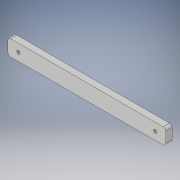
# Autodesk Inventor part: Fourbar-Coupler
Saved by Autodesk Inventor 2019 (Build 230136000, 136)
## iProperties
Created: 2021-06-06
Part Number: Fourbar-Coupler
Material: Generic
Document SubType Name: Modeling
Designer: micha
Density: 1 g/cm^3
Appearance: Default
Author: micha
Autodesk Inventor part; units mm, degrees
ref_plane "YZ Plane" through (0, 0, 0) normal (1, 0, 0) x (0, 1, 0)
ref_plane "XZ Plane" through (0, 0, 0) normal (0, 1, 0) x (-1, 0, 0)
ref_plane "XY Plane" through (0, 0, 0) normal (0, 0, 1) x (1, 0, 0)
sketch "Sketch1" plane through (0, 0, 0) normal (0, 0, 1) x (1, 0, 0)
  line L0 (0, 0) -> (300, 0)
  line L1 (300, 0) -> (300, 30)
  line L2 (300, 30) -> (0, 30)
  line L3 (0, 30) -> (0, 0)
  dimension "d0" = 300
  dimension "d1" = 30
  constraints: 8 end point, 2 parallel, 1 horizontal, 1 perpendicular
  measures "d0" distance of L2.end L1.end
  measures "d1" distance of L1.end L0.end
extrude "Extrusion1" add sketch "Sketch1" along normal blind 12
fillet "Fillet1" radius 5 1 edges at (0, 30, 6)
fillet "Fillet2" radius 5 3 edges at (300, 30, 6) (300, 0, 6) (0, 0, 6)
sketch "Sketch2" plane through (0, 0, 12) normal (0, 0, 1) x (1, 0, 0)
  line L0 (0, 25) -> (0, 5) projected
  line L1 (0, 15) -> (20, 15)
  circle A0 centre (20, 15) radius 3
  line L2 (5, 0) -> (295, 0) projected
  line L3 (150, 0) -> (150, 30)
  line L4 (295, 30) -> (5, 30) projected
  circle A1 centre (280, 15) radius 3
  point P0 (0, 0)
  dimension "d6" = 20
  dimension "d7" = 6
  constraints: 4 end point, 3 midpoint, 2 centre point, 1 coincident, 1 horizontal, 1 symmetric about line, 1 other
  measures "d6" distance of L1.start L1.end
  measures "d7" diameter of A0
extrude "Extrusion2" cut sketch "Sketch2" against normal through all
body "Solid1"
